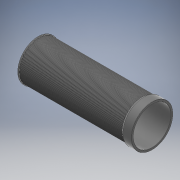
# Autodesk Inventor part: GuiderTube
Saved by Autodesk Inventor 2022 (Build 260153000, 153)
## iProperties
Created: 2021-05-10
Part Number: GuiderTube
Material: Generic
Document SubType Name: Modeling
Designer: Mick Veldhuis
Density: 1 g/cm^3
Appearance: Default
Author: Mick Veldhuis
Autodesk Inventor part; units mm, degrees
ref_plane "YZ Plane" through (0, 0, 0) normal (1, 0, 0) x (0, 1, 0)
ref_plane "XZ Plane" through (0, 0, 0) normal (0, 1, 0) x (-1, 0, 0)
sketch "Sketch3" plane through (0, 0, 0) normal (1, 0, 0) x (0, 1, 0)
  circle A0 centre (0, 0) radius 79
  constraints: 1 centre point, 1 coincident
extrude "Extrusion2" add sketch "Sketch3" along normal blind 4
sketch "Sketch4" plane through (4, 0, 0) normal (1, 0, 0) x (0, 0, -1)
  circle A0 centre (0, 0) radius 77
  circle A1 centre (0, 0) radius 73
  constraints: 2 centre point, 2 coincident
extrude "Extrusion3" add sketch "Sketch4" along normal blind 400
ref_plane "Work Plane1" through (404, 0, 0) normal (1, 0, 0) x (0, 0, -1)
sketch "Sketch5" plane through (404, 0, 0) normal (1, 0, 0) x (0, 0, -1)
  circle A0 centre (0, 0) radius 81
  circle A1 centre (0, 0) radius 73
  constraints: 2 centre point, 2 coincident
extrude "Extrusion4" add sketch "Sketch5" along normal blind 40
chamfer "Chamfer1" distance 4 angle 60 1 edges at (404, 0, 81) measured on face at (404, 0, 78.1669)
sketch "Sketch7" plane through (0, 0, 0) normal (-1, 0, 0) x (0, 0, 1)
  circle A0 centre (0, 0) radius 16
  circle A1 centre (0, 0) radius 40
  circle A2 centre (0, 0) radius 14
  constraints: 3 centre point, 2 coincident
extrude "Extrusion5" add sketch "Sketch7" along normal blind 20 contours A1
extrude "Extrusion6" add sketch "Sketch7" along normal blind 40 contours A0
fillet "Fillet1" radius 0.8 1 edges at (-40, 0, -16)
chamfer "Chamfer2" distance 8 angle 45 1 edges at (-20, 0, -40)
fillet "Fillet2" radius 1 2 edges at (444, 0, 81) (444, 0, 73)
extrude "Extrusion7" cut sketch "Sketch7" against normal through all contours A2
sketch "Sketch8" plane through (0, 0, 0) normal (-1, 0, 0) x (0, 0, 1)
  point P0 (0, 0)
body "Solid2"
